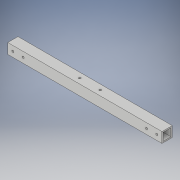
# Autodesk Inventor part: 17in 1x1 Beam
Saved by Autodesk Inventor 2018 (Build 220112000, 112)
## iProperties
Created: 2019-01-16
Part Number: 17in 1x1 Beam
Material: Generic
Document SubType Name: Modeling
Designer: Gabriel
Density: 1 g/cm^3
Appearance: Default
Author: Gabriel
Autodesk Inventor part; units mm, degrees
ref_plane "YZ Plane" through (0, 0, 0) normal (1, 0, 0) x (0, 1, 0)
ref_plane "XZ Plane" through (0, 0, 0) normal (0, 1, 0) x (-1, 0, 0)
ref_plane "XY Plane" through (0, 0, 0) normal (0, 0, 1) x (1, 0, 0)
sketch "Sketch1" plane through (0, 0, 0) normal (1, 0, 0) x (0, 1, 0)
  line L0 (4.2484, 4.9473) -> (-21.1516, 4.9473)
  line L1 (-21.1516, 4.9473) -> (-21.1516, -20.4527)
  line L2 (-21.1516, -20.4527) -> (4.2484, -20.4527)
  line L3 (4.2484, -20.4527) -> (4.2484, 4.9473)
  line L4 (1.0734, 1.7723) -> (-17.9766, 1.7723)
  line L5 (-17.9766, 1.7723) -> (-17.9766, -17.2777)
  line L6 (-17.9766, -17.2777) -> (1.0734, -17.2777)
  line L7 (1.0734, -17.2777) -> (1.0734, 1.7723)
  point P0 (0, 0)
  dimension "d0" = 25.4
  dimension "d1" = 25.4
  dimension "d2" = 3.175
  constraints: 16 end point, 4 parallel, 2 perpendicular, 1 horizontal, 3 other
  measures "d0" distance of L2.end L1.end
  measures "d1" distance of L1.end L0.end
  measures "d2" distance between parallel lines of L3 L7
extrude "Extrusion1" add sketch "Sketch1" along normal blind 381
sketch "Sketch2" plane through (0, -21.1516, -20.4527) normal (0, 0, -1) x (-1, 0, 0)
  line L0 (0, 0) -> (0, 25.4) construction
  line L1 (0, 12.7) -> (-12.7, 12.7) construction
  line L2 (-12.7, 12.7) -> (-38.1, 12.7) construction
  line L3 (-381, 0) -> (-381, 25.4) construction
  line L4 (-381, 12.7) -> (-368.3, 12.7) construction
  line L5 (-368.3, 12.7) -> (-342.9, 12.7) construction
  circle A0 centre (-368.3, 12.7) radius 2.5797
  circle A1 centre (-342.9, 12.7) radius 2.5797
  circle A2 centre (-12.7, 12.7) radius 2.5797
  circle A3 centre (-38.1, 12.7) radius 2.5797
  point P0 (0, 21.1516)
  dimension "d5" = 12.7
  dimension "d6" = 25.4
  dimension "d7" = 12.7
  dimension "d8" = 25.4
  dimension "d9" = 5.1594
  dimension "d10" = 5.1594
  dimension "d11" = 5.1594
  dimension "d12" = 5.1594
  constraints: 8 end point, 4 centre point, 4 coincident, 2 horizontal, 2 midpoint, 2 point on line
  measures "d5" distance of L1.start L1.end
  measures "d6" distance of L1.end L2.end
  measures "d7" distance of L4.start L4.end
  measures "d8" distance of L4.end L5.end
  measures "d9" diameter of A0
  measures "d10" diameter of A1
  measures "d11" diameter of A2
  measures "d12" diameter of A3
extrude "Extrusion2" cut sketch "Sketch2" against normal blind 431.8
sketch "Sketch3" plane through (0, 4.2484, 4.9473) normal (0, 1, 0) x (1, 0, 0)
  line L0 (0, 25.4) -> (381, 25.4) construction
  line L1 (190.5, 25.4) -> (190.5, 12.7) construction
  line L2 (190.5, 25.4) -> (203.2, 25.4) construction
  line L3 (190.5, 12.7) -> (215.9, 12.7) construction
  line L4 (215.9, 12.7) -> (165.1, 12.7) construction
  circle A0 centre (165.1, 12.7) radius 2.5797
  circle A1 centre (215.9, 12.7) radius 2.5797
  point P0 (0, 4.9473)
  dimension "d15" = 12.7
  dimension "d16" = 90
  dimension "d17" = 25.4
  dimension "d18" = 50.8
  dimension "d19" = 5.1594
  constraints: 8 end point, 2 centre point, 2 coincident, 2 horizontal, 1 midpoint, 1 perpendicular, 1 point on line, 1 vertical
  measures "d15" distance of L1.start L1.end
  measures "d16" angle of L1 L2
  measures "d17" distance of L1.end L3.end
  measures "d18" distance of L3.end L4.end
  measures "d19" diameter of A0
extrude "Extrusion3" cut sketch "Sketch3" against normal blind 77.7875
body "Solid1"
